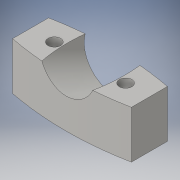
# Autodesk Inventor part: wedgeBlock
Saved by Autodesk Inventor 2016 (Build 200138000, 138)
## iProperties
Created: 2016-01-13
Part Number: wedgeBlock
Material: Generic
Document SubType Name: Modeling
Designer: ddeboer
Density: 1 g/cm^3
Appearance: Default
Author: ddeboer
Autodesk Inventor part; units mm, degrees
ref_plane "YZ Plane" through (0, 0, 0) normal (1, 0, 0) x (0, 1, 0)
ref_plane "XZ Plane" through (0, 0, 0) normal (0, 1, 0) x (-1, 0, 0)
ref_plane "XY Plane" through (0, 0, 0) normal (0, 0, 1) x (1, 0, 0)
sketch "Sketch1" plane through (0, 0, 0) normal (0, 1, 0) x (-1, 0, 0)
  line L0 (0, 0) -> (63.5, 0)
  line L1 (63.5, 0) -> (63.5, -25.4)
  line L2 (63.5, -25.4) -> (0, -25.4)
  line L3 (0, -25.4) -> (0, 0)
  dimension "d0" = 63.5
  dimension "d1" = 25.4
  constraints: 8 end point, 2 parallel, 1 horizontal, 1 perpendicular
  measures "d0" distance of L1.end L2.end
  measures "d1" distance of L2.end L0.start
extrude "Extrusion1" add sketch "Sketch1" along normal blind 26.1938
sketch "Sketch2" plane through (0, 0, 0) normal (0, -1, 0) x (1, 0, 0)
  line L0 (-63.5, 0) -> (0, 0) projected
  line L1 (-31.75, 0) -> (-31.75, -25.4) construction
  line L2 (0, -25.4) -> (-63.5, -25.4) projected
  circle A0 centre (-50.8, -12.7) radius 4.7004
  circle A1 centre (-12.7, -12.7) radius 4.7004
  dimension "d4" = 19.05
  dimension "d5" = 12.7
  constraints: 2 centre point, 2 end point, 2 midpoint, 1 symmetric about line, 1 other
  measures "d4" distance from line of L1 A0.centre
  measures "d5" distance from line of A0.centre L0
hole "Hole1" at (-12.7, 0, -12.7) at (-50.8, 0, -12.7) direction (0, 1, 0) diameter 6.7564 end through all clearance for "Flat Head Machine Screw (82)" size "1/4" standard "Ansi Unified Screw Threads"
ref_plane "Work Plane6" through (-63.5, 25.0611, -27.764) normal (0, -0.4321, -0.9018) x (-1, 0, 0)
ref_plane "Work Plane5" through (-63.5, 26.1938, -25.4) normal (0, -0.4321, -0.9018) x (-1, 0, 0)
sketch "Sketch10" plane through (-63.5, 25.0611, -27.764) normal (0, -0.4321, -0.9018) x (-1, 0, 0)
  circle A0 centre (-31.75, -4.826) radius 15.113
  line L0 (-63.5, 0) -> (0, 0) projected
  point P0 (-63.5, -34.5974)
  dimension "d50" = 30.226
  dimension "d51" = 4.826
  constraints: 1 centre point
  measures "d50" diameter of A0
  measures "d51" distance from line of A0.centre L0
extrude "Extrusion9" cut sketch "Sketch10" along normal mid plane 76.2
sketch "Sketch6" plane through (0, 0, 0) normal (0, -1, 0) x (1, 0, 0)
  line L0 (0, 0) -> (-63.5, 0) projected
  circle A0 centre (-31.75, -165.1) radius 165.1
  line L1 (-63.5, -25.4) -> (-63.5, 0) projected
  line L2 (-63.5, 0) -> (-63.5, -3.0816)
  line L3 (0, 0) -> (0, -3.0816)
  line L4 (0, 0) -> (0, -25.4) projected
  dimension "d28" = 330.2
  dimension "d29" = 165.1
  constraints: 4 end point, 2 point on circle, 2 point on line, 1 centre point
  measures "d28" diameter of A0
  measures "d29" distance from line of L0 A0.centre
extrude "Extrusion5" cut sketch "Sketch6" against normal blind 50.8 contours L3 A0 L0 | A0 L1 L0
sketch "Sketch7" plane through (0, 0, 0) normal (0, -1, 0) x (1, 0, 0)
  line L0 (-63.5, -25.4) -> (0, -25.4) construction
  line L1 (-31.75, -25.4) -> (-31.75, 139.7) construction
  line L2 (-31.75, -25.4) -> (133.35, -25.4) construction
  circle A0 centre (-31.75, 139.7) radius 165.1
  line L3 (0, 0) -> (0, -25.4) projected
  line L4 (0, -22.3184) -> (0, -25.4)
  line L5 (0, -25.4) -> (-63.5, -25.4)
  line L6 (-63.5, -25.4) -> (-63.5, -22.3184)
  line L7 (-63.5, -25.4) -> (-63.5, 0) projected
  point P0 (0, -3.0816)
  point P1 (-63.5, -3.0816)
  dimension "d32" = 165.1
  dimension "d33" = 90
  constraints: 10 end point, 3 point on circle, 2 collinear, 2 point on line, 1 centre point, 1 coincident, 1 horizontal, 1 midpoint, 1 perpendicular, 1 vertical
  measures "d32" distance of L1.start L1.end
  measures "d33" angle of L2 L1
extrude "Extrusion6" cut sketch "Sketch7" against normal blind 50.8 contours A0 L5 L6 | L3 L5 A0
sketch "Sketch11" plane through (0, 26.1938, 0) normal (0, 1, 0) x (1, 0, 0)
  line L0 (8.9616, -13.4203) -> (-66.3152, -13.4203)
  line L1 (-66.3152, -13.4203) -> (-66.3152, 46.0555)
  line L2 (-66.3152, 46.0555) -> (8.9616, 46.0555)
  line L3 (8.9616, 46.0555) -> (8.9616, -13.4203)
  point P0 (0, 0)
  constraints: 8 end point, 2 parallel, 1 horizontal, 1 perpendicular
extrude "Extrusion10" cut sketch "Sketch11" against normal blind 0.7937
body "Solid1"
